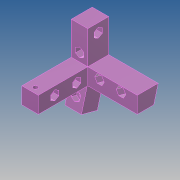
# Autodesk Inventor part: KB33-046-004-013 - Уголок
Saved by Autodesk Inventor 2020 (Build 240168000, 168)
## iProperties
Created: 2021-06-26
Part Number: KB33-046-004-013 - Уголок
Material: Пластик АБС
Document SubType Name: Modeling
Designer: Петров Иван
Mass: 37.7536 g
Surface Area: 125.462 cm^2
Volume: 35.6166 cm^3
Density: 1.06 g/cm^3
Appearance: Гладкий — пурпурный
Author: Петров Иван
Autodesk Inventor part; units mm, degrees
ref_plane "YZ Plane" through (0, 0, 0) normal (1, 0, 0) x (0, 1, 0)
ref_plane "XZ Plane" through (0, 0, 0) normal (0, 1, 0) x (-1, 0, 0)
sketch "Эскиз1" plane through (0, 0, 0) normal (0, 1, 0) x (-1, 0, 0)
  line L0 (0, 0) -> (0, -15)
  line L1 (0, -15) -> (60, -15)
  line L2 (60, -15) -> (60, 0)
  line L3 (60, 0) -> (0, 0)
  line L4 (0, -15) -> (15, -15)
  line L5 (15, -15) -> (15, 45)
  line L6 (15, 45) -> (0, 45)
  line L7 (0, 45) -> (0, -15)
  point P0 (15, 0)
  dimension "d0" = 60
  dimension "d1" = 15
  dimension "d2" = 15
  dimension "d3" = 60
  constraints: 16 end point, 4 parallel, 2 perpendicular, 1 point on line, 1 vertical
  measures "d0" distance of L1.end L0.end
  measures "d1" distance of L1.end L2.end
  measures "d2" distance of L0.end L4.end
  measures "d3" distance of L5.end L4.end
extrude "Выдавливание1" add sketch "Эскиз1" along normal blind 15
draft "НаклГрань1" angle 15 pull direction (0, -1, 0) faces at (0, 5, -5) fixed edges at (0, 0, -7.5)
sketch "Эскиз3" plane through (0, 0, 45) normal (0.9659258, -0.258819, 0) x (0, 0, -1)
  line L0 (0, 15.5291) -> (60, 15.5291) projected
  line L1 (45, 15.5291) -> (60, 15.5291)
  line L2 (60, 15.5291) -> (60, -24.4709)
  line L3 (60, -24.4709) -> (45, -24.4709)
  line L4 (45, -24.4709) -> (45, 15.5291)
  point P0 (45, 0)
  point P1 (60, 15.5291)
  dimension "d9" = 40
  dimension "d14" = 15
  constraints: 8 end point, 2 parallel, 1 horizontal, 1 perpendicular, 1 point on line
  measures "d9" distance of L1.end L2.end
  measures "d14" distance of L2.end L3.end
extrude "Выдавливание2" add sketch "Эскиз3" against normal blind 15
sketch "Эскиз4" plane through (0, 15, 0) normal (0, 1, 0) x (1, 0, 0)
  line L0 (-15, 0) -> (0, 0) projected
  line L1 (4.0192, 0) -> (4.0192, 15) projected
  line L2 (-15, 0) -> (4.0192, 0)
  line L3 (4.0192, 0) -> (4.0192, 15)
  line L4 (4.0192, 15) -> (-15, 15)
  line L5 (-15, 15) -> (-15, 0)
  constraints: 8 end point, 2 parallel, 1 horizontal, 1 perpendicular
extrude "Выдавливание3" add sketch "Эскиз4" along normal blind 30
sketch "Эскиз7" plane through (-60, 0, 0) normal (0, 0, 1) x (1, 0, 0)
  line L0 (0, 0) -> (0, 15) projected
  line L1 (0, 7.5) -> (45, 7.5) construction
  circle A0 centre (15, 7.5) radius 2
  circle A1 centre (35, 7.5) radius 2
  point P0 (60, 0)
  dimension "d24" = 4
  dimension "d25" = 4
  dimension "d26" = 20
  dimension "d27" = 15
  constraints: 2 centre point, 2 end point, 2 point on line, 1 midpoint
  measures "d24" diameter of A0
  measures "d25" diameter of A1
  measures "d26" distance of A1.centre A0.centre
  measures "d27" distance from line of L0 A0.centre
extrude "Выдавливание6" cut sketch "Эскиз7" against normal through all
sketch "Эскиз8" plane through (-60, 0, 0) normal (0, 0, 1) x (1, 0, 0)
  circle A0 centre (15, 7.5) radius 2 projected
  line L0 (15, 11.8301) -> (18.75, 9.6651)
  line L1 (18.75, 9.6651) -> (18.75, 5.3349)
  line L2 (18.75, 5.3349) -> (15, 3.1699)
  line L3 (15, 3.1699) -> (11.25, 5.3349)
  line L4 (11.25, 5.3349) -> (11.25, 9.6651)
  line L5 (11.25, 9.6651) -> (15, 11.8301)
  circle A1 centre (35, 7.5) radius 2 projected
  line L6 (35, 11.8301) -> (38.75, 9.6651)
  line L7 (38.75, 9.6651) -> (38.75, 5.3349)
  line L8 (38.75, 5.3349) -> (35, 3.1699)
  line L9 (35, 3.1699) -> (31.25, 5.3349)
  line L10 (31.25, 5.3349) -> (31.25, 9.6651)
  line L11 (31.25, 9.6651) -> (35, 11.8301)
  line L12 (0, 0) -> (0, 15) projected
  point P0 (60, 0)
  dimension "d30" = 7.5
  constraints: 24 end point, 2 coincident, 1 horizontal alignment, 1 parallel, 26 other
  measures "d30" distance between parallel lines of L1 L4
extrude "Выдавливание7" cut sketch "Эскиз8" against normal blind 5
sketch "Эскиз9" plane through (-14.4889, 3.8823, 45) normal (-0.9659258, 0.258819, 0) x (0, 0, 1)
  circle A0 centre (-52.5, -14.4709) radius 2
  line L0 (-45, -24.4709) -> (-45, -4.0192) projected
  line L1 (-60, -24.4709) -> (-45, -24.4709) projected
  point P0 (-45, 0)
  dimension "d33" = 4
  dimension "d34" = 7.5
  dimension "d35" = 10
  constraints: 1 centre point
  measures "d33" diameter of A0
  measures "d34" distance from line of L0 A0.centre
  measures "d35" distance from line of L1 A0.centre
extrude "Выдавливание8" cut sketch "Эскиз9" against normal through all
sketch "Эскиз10" plane through (-14.4889, 3.8823, 45) normal (-0.9659258, 0.258819, 0) x (0, 0, 1)
  circle A0 centre (-52.5, -14.4709) radius 2 projected
  line L0 (-52.5, -10.1407) -> (-48.75, -12.3058)
  line L1 (-48.75, -12.3058) -> (-48.75, -16.6359)
  line L2 (-48.75, -16.6359) -> (-52.5, -18.801)
  line L3 (-52.5, -18.801) -> (-56.25, -16.6359)
  line L4 (-56.25, -16.6359) -> (-56.25, -12.3058)
  line L5 (-56.25, -12.3058) -> (-52.5, -10.1407)
  line L6 (-45, -24.4709) -> (-45, -4.0192) projected
  point P0 (-45, 0)
  dimension "d38" = 7.5
  constraints: 12 end point, 1 coincident, 1 parallel, 13 other
  measures "d38" distance between parallel lines of L4 L1
extrude "Выдавливание9" cut sketch "Эскиз10" against normal blind 5 contours A0 | L0 L1 L2 L3 L4 L5
sketch "Эскиз11" plane through (0, 0, 45) normal (0.9659258, -0.258819, 0) x (0, 0, -1)
  line L0 (0, 0) -> (0, 15.5291) projected
  line L1 (0, -3.8823) -> (0, 10.6066) projected
  line L2 (0, 6) -> (60, 6) construction
  line L3 (0, 0) -> (45, 0) projected
  circle A0 centre (14.8012, 6) radius 2
  circle A1 centre (34.3241, 6) radius 2
  dimension "d41" = 6
  dimension "d42" = 4
  dimension "d43" = 4
  constraints: 3 point on line, 2 centre point, 2 end point, 1 horizontal
  measures "d41" distance between parallel lines of L3 L2
  measures "d42" diameter of A0
  measures "d43" diameter of A1
extrude "Выдавливание10" cut sketch "Эскиз11" against normal through all
ref_plane "РабПлоскость1" through (-22.2163, 5.9528, 45) normal (0.9659258, -0.258819, 0) x (0, 0, -1)
sketch "Эскиз12" plane through (-22.2163, 5.9528, 45) normal (0.9659258, -0.258819, 0) x (0, 0, -1)
  circle A0 centre (34.3241, 6) radius 2 projected
  line L0 (36.4892, 9.75) -> (38.6543, 6)
  line L1 (38.6543, 6) -> (36.4892, 2.25)
  line L2 (36.4892, 2.25) -> (32.1591, 2.25)
  line L3 (32.1591, 2.25) -> (29.994, 6)
  line L4 (29.994, 6) -> (32.1591, 9.75)
  line L5 (32.1591, 9.75) -> (36.4892, 9.75)
  circle A1 centre (14.8012, 6) radius 2 projected
  line L6 (12.6361, 9.75) -> (16.9663, 9.75)
  line L7 (16.9663, 9.75) -> (19.1313, 6)
  line L8 (19.1313, 6) -> (16.9663, 2.25)
  line L9 (16.9663, 2.25) -> (12.6361, 2.25)
  line L10 (12.6361, 2.25) -> (10.4711, 6)
  line L11 (10.4711, 6) -> (12.6361, 9.75)
  line L12 (45, 10.6066) -> (0, 10.6066) projected
  point P0 (45, 0)
  dimension "d47" = 7.5
  dimension "d48" = 7.5
  constraints: 24 end point, 2 coincident, 2 parallel, 26 other
  measures "d47" distance between parallel lines of L2 L5
  measures "d48" distance between parallel lines of L9 L6
extrude "Выдавливание11" cut sketch "Эскиз12" along normal blind 15 contours A0 | L0 L1 L2 L3 L4 L5 | A1 | L6 L7 L8 L9 L10 L11
sketch "Эскиз13" plane through (-15, 15, -15) normal (-1, 0, 0) x (0, 0, 1)
  circle A0 centre (7.5, 7.5) radius 2
  line L0 (0, 0) -> (0, 30) projected
  line L1 (0, 0) -> (15, 0) projected
  point P0 (15, -15)
  dimension "d51" = 4
  dimension "d52" = 7.5
  dimension "d53" = 7.5
  constraints: 1 centre point
  measures "d51" diameter of A0
  measures "d52" distance from line of L0 A0.centre
  measures "d53" distance from line of A0.centre L1
extrude "Выдавливание12" cut sketch "Эскиз13" against normal blind 34.75
sketch "Эскиз14" plane through (-15, 15, -15) normal (-1, 0, 0) x (0, 0, 1)
  circle A0 centre (7.5, 7.5) radius 2 projected
  line L0 (7.5, 11.8301) -> (11.25, 9.6651)
  line L1 (11.25, 9.6651) -> (11.25, 5.3349)
  line L2 (11.25, 5.3349) -> (7.5, 3.1699)
  line L3 (7.5, 3.1699) -> (3.75, 5.3349)
  line L4 (3.75, 5.3349) -> (3.75, 9.6651)
  line L5 (3.75, 9.6651) -> (7.5, 11.8301)
  point P0 (15, -15)
  dimension "d56" = 7.5
  constraints: 12 end point, 1 coincident, 13 other
  measures "d56" distance between parallel lines of L1 L4
extrude "Выдавливание13" cut sketch "Эскиз14" against normal blind 6 contours A0 | L0 L1 L2 L3 L4 L5
sketch "Эскиз15" plane through (-15, 15, 0) normal (0, 0, 1) x (1, 0, 0)
  circle A0 centre (9.5, 22) radius 2
  line L0 (0, 0) -> (0, 30) projected
  line L1 (0, 30) -> (19.0192, 30) projected
  point P0 (15, -15)
  dimension "d59" = 4
  dimension "d60" = 9.5
  dimension "d66" = 8
  constraints: 1 centre point
  measures "d59" diameter of A0
  measures "d60" distance from line of L0 A0.centre
  measures "d66" distance from line of L1 A0.centre
extrude "Выдавливание14" cut sketch "Эскиз15" against normal through all
sketch "Эскиз16" plane through (-15, 15, 0) normal (0, 0, 1) x (1, 0, 0)
  circle A0 centre (9.5, 22) radius 2 projected
  line L0 (9.5, 26.3301) -> (13.25, 24.1651)
  line L1 (13.25, 24.1651) -> (13.25, 19.8349)
  line L2 (13.25, 19.8349) -> (9.5, 17.6699)
  line L3 (9.5, 17.6699) -> (5.75, 19.8349)
  line L4 (5.75, 19.8349) -> (5.75, 24.1651)
  line L5 (5.75, 24.1651) -> (9.5, 26.3301)
  point P0 (15, -15)
  dimension "d63" = 7.5
  constraints: 12 end point, 1 coincident, 13 other
  measures "d63" distance between parallel lines of L1 L4
extrude "Выдавливание15" cut sketch "Эскиз16" against normal blind 6
sketch "Эскиз17" plane through (0, 15, 0) normal (0, 1, 0) x (1, 0, 0)
  circle A0 centre (-55, 7.5) radius 2
  line L0 (-60, 0) -> (-15, 0) projected
  line L1 (-60, 15) -> (-60, 0) projected
  point P0 (0, 0)
  dimension "d78" = 4
  dimension "d79" = 7.5
  dimension "d80" = 5
  constraints: 1 centre point
  measures "d78" diameter of A0
  measures "d79" distance from line of L0 A0.centre
  measures "d80" distance from line of L1 A0.centre
extrude "Выдавливание16" cut sketch "Эскиз17" against normal through all
sketch "Эскиз18" plane through (0, 0, 0) normal (0, -1, 0) x (1, 0, 0)
  circle A0 centre (-55, -7.5) radius 2 projected
  line L0 (-55, -3.1699) -> (-51.25, -5.3349)
  line L1 (-51.25, -5.3349) -> (-51.25, -9.6651)
  line L2 (-51.25, -9.6651) -> (-55, -11.8301)
  line L3 (-55, -11.8301) -> (-58.75, -9.6651)
  line L4 (-58.75, -9.6651) -> (-58.75, -5.3349)
  line L5 (-58.75, -5.3349) -> (-55, -3.1699)
  line L6 (-60, -15) -> (-60, 0) projected
  point P0 (0, 0)
  dimension "d83" = 7.5
  constraints: 12 end point, 1 coincident, 1 parallel, 13 other
  measures "d83" distance between parallel lines of L1 L4
extrude "Выдавливание17" cut sketch "Эскиз18" against normal blind 5
equation "\"d48\" = d47"
